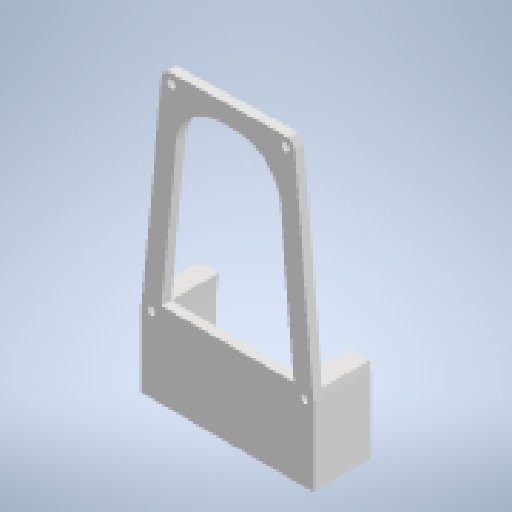
# Autodesk Inventor part: holder
Saved by Autodesk Inventor 2023 (Build 270158000, 158)
## iProperties
Created: 2023-11-04
Part Number: holder
Material: Générique
Document SubType Name: Modeling
Designer: eleves
Density: 1 g/cm^3
Appearance: Par défaut
Author: eleves
Autodesk Inventor part; units mm, degrees
ref_plane "YZ Plane" through (0, 0, 0) normal (1, 0, 0) x (0, 1, 0)
ref_plane "XZ Plane" through (0, 0, 0) normal (0, 1, 0) x (-1, 0, 0)
ref_plane "XY Plane" through (0, 0, 0) normal (0, 0, 1) x (1, 0, 0)
sketch "Esquisse1" plane through (0, 0, 0) normal (0, 0, 1) x (1, 0, 0)
  circle A0 centre (-5.13, -4.2) radius 1.738 projected
  circle A1 centre (43.13, -2.93) radius 1.738 projected
  circle A2 centre (10.11, -55) radius 1.738 projected
  circle A3 centre (51.1638, -91.424) radius 1.5682 projected
  circle A4 centre (-13.5548, -91.424) radius 1.5682 projected
  line L0 (-5.13, -4.2) -> (43.13, -2.93) construction
  line L1 (-5.0248, -8.1986) -> (43.2352, -6.9286)
  line L2 (43.0248, 1.0686) -> (-5.2352, -0.2014)
  arc A5 (-5.2352, -0.2014) -> (-5.0248, -8.1986) centre (-5.13, -4.2) ccw
  arc A6 (43.2352, -6.9286) -> (43.0248, 1.0686) centre (43.13, -2.93) ccw
  arc A7 (-1.2987, -3.0506) -> (-8.9613, -5.3494) centre (-5.13, -4.2) ccw
  arc A8 (46.508, -5.0722) -> (39.752, -0.7878) centre (43.13, -2.93) ccw
  arc A9 (-16.909, -89.2447) -> (-10.2005, -93.6032) centre (-13.5548, -91.424) ccw
  arc A10 (48.5091, -94.4161) -> (53.8185, -88.4319) centre (51.1638, -91.424) ccw
  line L3 (43.13, -2.93) -> (51.1638, -91.424) construction
  line L4 (39.1464, -3.2916) -> (47.1802, -91.7856)
  line L5 (55.1474, -91.0623) -> (47.1136, -2.5684)
  arc A11 (47.1136, -2.5684) -> (39.1464, -3.2916) centre (43.13, -2.93) ccw
  arc A12 (47.1802, -91.7856) -> (55.1474, -91.0623) centre (51.1638, -91.424) ccw
  line L6 (-5.13, -4.2) -> (-13.5548, -91.424) construction
  line L7 (-1.1485, -4.5846) -> (-9.5733, -91.8085)
  line L8 (-17.5362, -91.0394) -> (-9.1115, -3.8154)
  arc A13 (-1.1485, -4.5846) -> (-9.1115, -3.8154) centre (-5.13, -4.2) ccw
  arc A14 (-17.5362, -91.0394) -> (-9.5733, -91.8085) centre (-13.5548, -91.424) ccw
  line L9 (-13.5548, -91.424) -> (51.1638, -91.424) construction
  line L10 (-13.5548, -95.424) -> (51.1638, -95.424)
  line L11 (51.1638, -87.424) -> (-13.5548, -87.424)
  arc A15 (-13.5548, -87.424) -> (-13.5548, -95.424) centre (-13.5548, -91.424) ccw
  arc A16 (51.1638, -95.424) -> (51.1638, -87.424) centre (51.1638, -91.424) ccw
  point P0 (0, 0)
  point P1 (19, -3.565)
  point P2 (2.49, -29.6)
  point P3 (-1.7224, -73.212)
  point P4 (30.6369, -73.212)
  point P5 (47.1469, -47.177)
  point P6 (-9.3424, -47.812)
  point P7 (18.8045, -91.424)
  point P8 (39.4855, -7.0273)
  point P9 (46.7842, -87.424)
  point P10 (-9.1498, -87.424)
  point P11 (-1.4886, -8.1056)
  point P12 (-9.1115, -3.8154)
  point P13 (51.1638, -95.424)
  point P14 (47.1136, -2.5684)
  dimension "d2" = 8
  dimension "d3" = 8
  dimension "d5" = 8
  dimension "d6" = 8
  constraints: 32 end point, 24 point on circle, 16 tangent, 12 centre point, 4 midpoint, 4 parallel, 1 horizontal
  measures "d2" distance between parallel lines of L2 L1
  measures "d3" distance between parallel lines of L7 L8
  measures "d5" distance between parallel lines of L5 L4
  measures "d6" distance between parallel lines of L10 L11
extrude "Extrusion1" add sketch "Esquisse1" along normal blind 4 contours A5 A7 A13 L7 L1 | L1 L7 L11 A15 A9 L8 A5 | L7 A13 A7 L2 A8 A11 L4 L1 | L4 A11 A8 A6 L1 | L1 A6 L5 A10 A16 L11 L4 | L11 L4 A12 A10 L10 A9 A14 L7 | L7 A14 A9 A15 L11 | L11 A16 A10 A12 L4
fillet "Congé1" radius 19 2 edges at (-1.4886, -8.1056, 2) (39.4855, -7.0273, 2)
sketch "Esquisse2" plane through (0, 0, 0) normal (0, 0, -1) x (-1, 0, 0)
  arc A0 (9.1115, -3.8154) -> (5.2352, -0.2014) centre (5.13, -4.2) ccw projected
  line L0 (-43.0248, 1.0686) -> (5.2352, -0.2014) projected
  arc A1 (-43.0248, 1.0686) -> (-47.1136, -2.5684) centre (-43.13, -2.93) ccw projected
  line L1 (-55.1474, -91.0623) -> (-47.1136, -2.5684) projected
  arc A2 (-55.1474, -91.0623) -> (-51.1638, -95.424) centre (-51.1638, -91.424) ccw projected
  line L2 (13.5548, -95.424) -> (-51.1638, -95.424) projected
  arc A3 (13.5548, -95.424) -> (17.5362, -91.0394) centre (13.5548, -91.424) ccw projected
  line L3 (9.1115, -3.8154) -> (17.5362, -91.0394) projected
  arc A4 (-21.6744, -7.496) -> (-41.0964, -24.7716) centre (-22.1742, -26.4894) ccw projected
  line L4 (-15.3081, -7.6635) -> (-21.6744, -7.496) projected
  arc A5 (3.104, -24.8303) -> (-15.3081, -7.6635) centre (-15.808, -26.657) ccw projected
  line L5 (9.1498, -87.424) -> (3.104, -24.8303) projected
  line L6 (-46.7842, -87.424) -> (9.1498, -87.424) projected
  line L7 (-41.0964, -24.7716) -> (-46.7842, -87.424) projected
  circle A6 centre (5.13, -4.2) radius 1.738 projected
  circle A7 centre (13.5548, -91.424) radius 1.5682 projected
  circle A8 centre (-43.13, -2.93) radius 1.738 projected
  circle A9 centre (-51.1638, -91.424) radius 1.5682 projected
  line L8 (-41.0964, -24.7716) -> (-46.7842, -87.424) projected
  line L9 (-46.7842, -87.424) -> (-47.5105, -95.424)
  line L10 (-55.1474, -91.0623) -> (-47.1136, -2.5684) projected
  line L11 (-46.7842, -87.424) -> (9.1498, -87.424) projected
  line L12 (-46.7842, -87.424) -> (-54.8171, -87.424)
  line L13 (9.1498, -87.424) -> (9.9225, -95.424)
  line L14 (9.1498, -87.424) -> (17.187, -87.424)
  point P0 (0, 0)
  constraints: 8 end point, 4 collinear, 4 point on line
extrude "Extrusion2" add sketch "Esquisse2" along normal blind 20 contours L3 A3 L2 L13 L14 | L9 L2 A2 L1 L12
sketch "Esquisse3" plane through (-13.5548, -95.424, 4) normal (0, -1, 0) x (1, 0, 0)
  line L0 (3.6323, -4) -> (61.0652, -4) projected
  line L1 (61.0652, -4) -> (61.0652, -24) projected
  line L2 (64.7185, -24) -> (61.0652, -24) projected
  line L3 (64.7185, -24) -> (64.7185, 0) projected
  line L4 (0, 0) -> (64.7185, 0) projected
  line L5 (0, -24) -> (0, 0) projected
  line L6 (3.6323, -24) -> (0, -24) projected
  line L7 (3.6323, -4) -> (3.6323, -24) projected
  line L8 (0, -24) -> (0, 0) projected
  line L9 (-3.9815, 0) -> (0, 0) projected
  line L10 (-3.9815, -24) -> (-3.9815, 0) projected
  line L11 (0, -24) -> (-3.9815, -24) projected
  line L12 (68.7022, -24) -> (68.7022, 0) projected
  line L13 (64.7185, 0) -> (68.7022, 0) projected
  line L14 (64.7185, -24) -> (64.7185, 0) projected
  line L15 (68.7022, -24) -> (64.7185, -24) projected
  point P0 (13.5548, -4)
  point P1 (0, 0)
  point P2 (64.7185, 0)
extrude "Extrusion3" add sketch "Esquisse3" along normal blind 25
sketch "Esquisse4" plane through (0, 0, 4) normal (0, 0, 1) x (1, 0, 0)
  arc A0 (-5.2352, -0.2014) -> (-9.1115, -3.8154) centre (-5.13, -4.2) ccw projected
  line L0 (-9.1115, -3.8154) -> (-17.5362, -91.0394) projected
  arc A1 (-17.5362, -91.0394) -> (-13.5548, -95.424) centre (-13.5548, -91.424) ccw projected
  line L1 (-13.5548, -95.424) -> (-17.5362, -95.424) projected
  line L2 (-17.5362, -95.424) -> (-17.5362, -120.424) projected
  line L3 (55.1474, -120.424) -> (-17.5362, -120.424) projected
  line L4 (55.1474, -95.424) -> (55.1474, -120.424) projected
  line L5 (55.1474, -95.424) -> (51.1638, -95.424) projected
  arc A2 (51.1638, -95.424) -> (55.1474, -91.0623) centre (51.1638, -91.424) ccw projected
  line L6 (55.1474, -91.0623) -> (47.1136, -2.5684) projected
  arc A3 (47.1136, -2.5684) -> (43.0248, 1.0686) centre (43.13, -2.93) ccw projected
  line L7 (43.0248, 1.0686) -> (-5.2352, -0.2014) projected
  line L8 (41.0964, -24.7716) -> (46.7842, -87.424) projected
  line L9 (46.7842, -87.424) -> (-9.1498, -87.424) projected
  line L10 (-9.1498, -87.424) -> (-3.104, -24.8303) projected
  arc A4 (15.3081, -7.6635) -> (-3.104, -24.8303) centre (15.808, -26.657) ccw projected
  line L11 (15.3081, -7.6635) -> (21.6744, -7.496) projected
  arc A5 (41.0964, -24.7716) -> (21.6744, -7.496) centre (22.1742, -26.4894) ccw projected
  circle A6 centre (-5.13, -4.2) radius 1.738 projected
  circle A7 centre (-13.5548, -91.424) radius 1.5682 projected
  circle A8 centre (43.13, -2.93) radius 1.738 projected
  circle A9 centre (51.1638, -91.424) radius 1.5682 projected
  line L12 (-17.5362, -91.0394) -> (-17.187, -87.424) projected
  line L13 (-17.5362, -95.424) -> (-17.5362, -91.0394)
  line L14 (55.1474, -91.0623) -> (55.1474, -95.424)
  point P0 (0, 0)
  point P1 (55.1474, -91.7856)
  point P2 (-17.5362, -91.8085)
  constraints: 4 end point, 1 collinear
extrude "Extrusion4" add sketch "Esquisse4" against normal up to surface (24 mm away) contours A1 L1 L13 | L14 L5 A2
sketch "Esquisse5" plane through (-13.5548, -120.424, 4) normal (0, -1, 0) x (1, 0, 0)
  line L0 (68.7022, 0) -> (-3.9815, 0) projected
  line L1 (-3.9815, 0) -> (-3.9815, -24) projected
  line L2 (68.7022, 0) -> (-3.9815, 0)
  line L3 (-3.9815, 0) -> (-3.9815, -24)
  line L4 (-3.9815, -24) -> (68.7022, -24)
  line L5 (68.7022, -24) -> (68.7022, 0)
  point P0 (13.5548, -4)
  constraints: 8 end point, 2 parallel, 1 horizontal, 1 perpendicular
extrude "Extrusion5" add sketch "Esquisse5" along normal blind 3
sketch "Esquisse6" plane through (-13.5548, -120.424, 4) normal (0, 1, 0) x (1, 0, 0)
  circle A0 centre (52.3133, 6.979) radius 1.6 projected
  circle A1 centre (52.3133, 16.979) radius 1.6 projected
  circle A2 centre (42.3133, 16.979) radius 1.6 projected
  circle A3 centre (42.3133, 6.979) radius 1.6 projected
  circle A4 centre (32.3133, 6.979) radius 1.6 projected
  circle A5 centre (32.3133, 16.979) radius 1.6 projected
  circle A6 centre (22.3133, 16.979) radius 1.6 projected
  circle A7 centre (22.3133, 6.979) radius 1.6 projected
  circle A8 centre (12.3133, 6.979) radius 1.6 projected
  circle A9 centre (12.3133, 16.979) radius 1.6 projected
  point P0 (13.5548, 4)
ref_plane "Plan de construction1" through (-33.0415, -128.424, -137.979) normal (0, -1, 0) x (1, 0, 0)
extrude "Extrusion6" cut sketch "Esquisse6" against normal up to surface (8 mm away)
